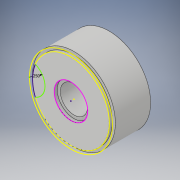
# Autodesk Inventor part: AutomobloxWheel
Saved by Autodesk Inventor 2018 (Build 220112000, 112)
## iProperties
Created: 2019-01-09
Part Number: AutomobloxWheel
Material: Generic
Document SubType Name: Modeling
Designer: 10043883
Density: 1 g/cm^3
Appearance: Default
Author: 10043883
Autodesk Inventor part; units mm, degrees
ref_plane "YZ Plane" through (0, 0, 0) normal (1, 0, 0) x (0, 1, 0)
ref_plane "XZ Plane" through (0, 0, 0) normal (0, 1, 0) x (-1, 0, 0)
ref_plane "XY Plane" through (0, 0, 0) normal (0, 0, 1) x (1, 0, 0)
sketch "Sketch1" plane through (0, 0, 0) normal (0, 0, 1) x (1, 0, 0)
  circle A0 centre (0, 0) radius 5.588
  circle A1 centre (0, 0) radius 6.858
  circle A2 centre (0, 0) radius 15.748
  circle A3 centre (0, 0) radius 17.018
  dimension "d0" = 11.176
  dimension "d1" = 1.27
  dimension "d2" = 8.89
  dimension "d3" = 1.27
  constraints: 4 centre point, 4 coincident
  measures "d0" diameter of A0
  measures "d1" radial gap between concentric circles of A0 A1
  measures "d2" radial gap between concentric circles of A1 A2
  measures "d3" radial gap between concentric circles of A2 A3
extrude "Extrusion1" add sketch "Sketch1" along normal blind 14.478
sketch "Sketch2" plane through (0, 0, 14.478) normal (0, 0, 1) x (1, 0, 0)
  circle A0 centre (0, 0) radius 5.588 projected
  circle A1 centre (0, 0) radius 6.858 projected
  circle A2 centre (0, 0) radius 15.748 projected
  circle A3 centre (0, 0) radius 17.018 projected
extrude "Extrusion2" add sketch "Sketch2" along normal blind 1.27 contours A2
sketch "Sketch4" plane through (0, 0, 14.478) normal (0, 0, 1) x (1, 0, 0)
  point P0 (0, 0)
sketch "Sketch5" plane through (0, 0, 15.748) normal (0, 0, 1) x (1, 0, 0)
  circle A0 centre (0, 0) radius 17.018 projected
  arc A1 (-10.668, 0) -> (-14.6107, 5.876) centre (-17.018, 0) ccw
  circle A2 centre (0, 0) radius 15.748 projected
  arc A3 (-14.6107, -5.876) -> (-10.668, 0) centre (-17.018, 0) ccw
  circle A4 centre (0, 0) radius 6.858 projected
  circle A5 centre (0, 0) radius 15.748 projected
  circle A6 centre (0, 0) radius 6.858 projected
  circle A7 centre (0, 0) radius 15.748 projected
  circle A8 centre (0, 0) radius 15.748 projected
  arc A9 (-14.6107, 5.876) -> (-14.6107, -5.876) centre (0, 0) ccw
  dimension "d9" = 6.35
  constraints: 8 point on circle, 3 centre point, 1 coincident, 1 concentric, 1 horizontal alignment, 3 other
  measures "d9" radius of A1
body "Solid1"
